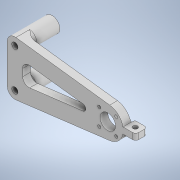
# Autodesk Inventor part: sensor_holder_1_mod
Saved by Autodesk Inventor 2020 (Build 240168000, 168)
## iProperties
Created: 2019-10-15
Part Number: sensor_holder_1_mod
Material: Generic
Document SubType Name: Modeling
Designer: psrob
Density: 1 g/cm^3
Appearance: Default
Author: psrob
Autodesk Inventor part; units mm, degrees
ref_plane "YZ Plane" through (0, 0, 0) normal (1, 0, 0) x (0, 1, 0)
ref_plane "XZ Plane" through (0, 0, 0) normal (0, 1, 0) x (-1, 0, 0)
ref_plane "XY Plane" through (0, 0, 0) normal (0, 0, 1) x (1, 0, 0)
sketch "Sketch1" plane through (0, 0, 0) normal (0, 0, 1) x (1, 0, 0)
  circle A0 centre (6, -12.5) radius 2
  circle A1 centre (6, 12.5) radius 2
  circle A2 centre (-10, -12.5) radius 2
  circle A3 centre (-10, 12.5) radius 2
  circle A4 centre (18, 0) radius 2.1
  circle A5 centre (28, 0) radius 2.1
  circle A6 centre (38, 0) radius 2.1
  circle A7 centre (50, 0) radius 6.5
  circle A8 centre (0, -12.5) radius 1.5
  circle A9 centre (0, 12.5) radius 1.5
  circle A10 centre (0, 0) radius 9
  line L0 (-6.52451, 22) -> (6.52451, 22)
  arc A11 (-8.148897, 20.972493) -> (-6.52451, 22) centre (-9.959763, 25.633047) ccw
  arc A12 (-8.148897, 20.972493) -> (-20.972493, 8.148897) centre (0, 0) ccw
  arc A13 (-22, 6.52451) -> (-20.972493, 8.148897) centre (-25.633047, 9.959763) ccw
  line L1 (-22, -6.52451) -> (-22, 6.52451)
  arc A14 (-20.972493, -8.148897) -> (-22, -6.52451) centre (-25.633047, -9.959763) ccw
  arc A15 (-20.972493, -8.148897) -> (-8.148897, -20.972493) centre (0, 0) ccw
  arc A16 (-6.52451, -22) -> (-8.148897, -20.972493) centre (-9.959763, -25.633047) ccw
  line L2 (6.52451, -22) -> (-6.52451, -22)
  arc A17 (8.148897, -20.972493) -> (6.52451, -22) centre (9.959763, -25.633047) ccw
  arc A18 (8.148897, -20.972493) -> (19.960204, -10.384615) centre (0, 0) ccw
  arc A19 (28.831406, -5) -> (19.960204, -10.384615) centre (28.831406, -15) ccw
  line L3 (28.831406, -5) -> (33.416876, -5)
  arc A20 (44.472292, -8.333333) -> (33.416876, -5) centre (33.416876, -25) ccw
  arc A21 (44.472292, -8.333333) -> (59.797959, -2) centre (50, 0) ccw
  arc A22 (33.416876, 5) -> (44.472292, 8.333333) centre (33.416876, 25) ccw
  line L4 (33.416876, 5) -> (28.831406, 5)
  arc A23 (19.960204, 10.384615) -> (28.831406, 5) centre (28.831406, 15) ccw
  arc A24 (19.960204, 10.384615) -> (8.148897, 20.972493) centre (0, 0) ccw
  arc A25 (6.52451, 22) -> (8.148897, 20.972493) centre (9.959763, 25.633047) ccw
  circle A26 centre (-10, -12.5) radius 5
  circle A27 centre (-10, 12.5) radius 5
  line L5 (66.5, 2) -> (66.5, -2)
  line L6 (66.5, 2) -> (59.797959, 2)
  arc A28 (59.797959, 2) -> (44.472292, 8.333333) centre (50, 0) ccw
  line L7 (59.797959, -2) -> (66.5, -2)
  dimension "d0" = 10
  dimension "d1" = 10
  constraints: 2 centre point, 2 coincident
  measures "d0" diameter of A26
  measures "d1" diameter of A27
extrude "Extrusion1" add sketch "Sketch1" along normal blind 20 contours A26 | A27
sketch "Sketch2" plane through (-10, -12.5, 20) normal (0, 0, 1) x (1, 0, 0)
  circle A0 centre (60, 12.5) radius 2.5
  circle A1 centre (60, 12.5) radius 10
  circle A2 centre (60, 12.5) radius 5
  circle A3 centre (0, 0) radius 5
  circle A4 centre (0, 0) radius 2
  circle A5 centre (0, 25) radius 5
  circle A6 centre (0, 25) radius 2
  line L0 (60, 12.5) -> (-0.617038, 4.96178)
  circle A7 centre (0, 0) radius 5
  line L1 (60, 12.5) -> (-0.617038, 20.03822)
  line L2 (0, 25) -> (-0.617038, 20.03822)
  line L3 (0, 0) -> (-0.617038, 4.96178)
  line L4 (61.234075, 2.576439) -> (0.617038, -4.96178)
  line L5 (0, 0) -> (0.617038, -4.96178)
  line L6 (60, 12.5) -> (61.234075, 2.576439)
  line L7 (61.234075, 22.423561) -> (0.617038, 29.96178)
  circle A8 centre (0, 25) radius 5
  line L8 (0, 25) -> (0.617038, 29.96178)
  line L9 (61.234075, 22.423561) -> (60, 12.5)
  point P0 (10, 12.5)
  point P1 (50.076439, 13.734075)
  point P2 (50.076439, 11.265925)
  point P3 (-0.617038, 4.96178)
  point P4 (0.617038, -4.96178)
  point P5 (0.617038, 29.96178)
  dimension "d4" = 20
  dimension "d5" = 10
  constraints: 20 end point, 6 perpendicular, 5 point on circle, 3 coincident, 2 centre point, 2 other
  measures "d4" diameter of A1
  measures "d5" diameter of A2
extrude "Extrusion2" add sketch "Sketch2" along normal blind 4 contours L9 A1 L6 A2 | A2 L1 A1 L9 | L6 A1 L0 A2 | A2 L0 A1 L1 | A1 L1 A5 L7 | L4 A3 L0 A1
sketch "Sketch3" plane through (0, 0, 20) normal (0, 0, 1) x (1, 0, 0)
  arc A0 (-10.617038, 7.53822) -> (-9.382962, 17.46178) centre (-10, 12.5) ccw
  arc A1 (-9.382962, 17.46178) -> (-10.617038, 7.53822) centre (-10, 12.5) ccw
  circle A2 centre (-10, 12.5) radius 2
  arc A3 (-9.382962, -17.46178) -> (-10.617038, -7.53822) centre (-10, -12.5) ccw
  arc A4 (-10.617038, -7.53822) -> (-9.382962, -17.46178) centre (-10, -12.5) ccw
  circle A5 centre (-10, -12.5) radius 2
  line L0 (-10, 12.5) -> (-15, 12.5)
  circle A6 centre (-10, 12.5) radius 5
  line L1 (-10, -12.5) -> (-15, -12.5)
  line L2 (-15, -12.5) -> (-15, 12.5)
  line L3 (-10, 12.5) -> (-5, 12.5)
  line L4 (-5, 12.5) -> (-5, -12.5)
  line L5 (-10, -12.5) -> (-5, -12.5)
  point P0 (0, 0)
  constraints: 12 end point, 4 point on circle, 3 perpendicular, 2 horizontal, 1 point on line
extrude "Extrusion3" add sketch "Sketch3" along normal blind 4 contours A1 L0 A2 L3 A0 | A0 L4 A3 A4 L2 A1 | L3 A2 L0 A1 A0 | L5 A5 L1 A4 A3 | A3 A4 L1 A5 L5
thicken "Thicken1" operation add thickness 1 both sides no extend neighbours yes toward (0, 0, -1) faces at (28.580011, -8.658994, 20)
thicken "Thicken2" operation add thickness 3 both sides no extend neighbours yes toward (-0.9953736, 0.0960805, 0) faces at (40.046264, 0.960805, 22.333333)
fillet "Fillet1" radius 4 2 edges at (-5, 6.8397, 21.5) (-5, -6.8397, 21.5)
fillet "Fillet2" radius 4 4 edges at (-10, 7.5, 19) (-6.2527, 15.8102, 19) (-6.2527, -15.8102, 19) (-10, -7.5, 19)
fillet "Fillet3" radius 2 2 edges at (37.0994, 1.6043, 21.5) (37.0994, -1.6043, 21.5)
sketch "Sketch4" plane through (0, 0, 0) normal (0, 1, 0) x (-1, 0, 0)
  line L0 (-51.234075, 19) -> (-51.234075, 19)
  line L1 (-51.234075, 19) -> (-51.234075, 24)
  line L2 (-51.234075, 24) -> (-51.234075, 24)
  line L3 (-51.234075, 19) -> (-51.234075, 24)
  line L4 (-51.234075, 24) -> (-60, 24)
  line L5 (-60, 24) -> (-68, 24)
  line L6 (-68, 24) -> (-68, 16.5)
  line L7 (-68, 16.5) -> (-60, 16.5)
  line L8 (-60, 16.5) -> (-60, 24)
  line L9 (-60, 24) -> (-57, 24)
  line L10 (-57, 24) -> (-57, 19)
  line L11 (-57, 19) -> (-60, 19)
  line L12 (-60, 19) -> (-60, 24)
  point P0 (0, 0)
  dimension "d17" = 8
  dimension "d18" = 7.5
  dimension "d19" = 3
  dimension "d20" = 5
  constraints: 16 end point, 4 parallel, 2 horizontal, 2 perpendicular
  measures "d17" distance of L7.end L6.end
  measures "d18" distance of L6.end L5.end
  measures "d19" distance of L10.end L11.end
  measures "d20" distance of L9.end L10.end
extrude "Extrusion4" add sketch "Sketch4" along normal mid plane 4
sketch "Sketch5" plane through (0, -2, 0) normal (0, -1, 0) x (1, 0, 0)
  line L0 (59.797959, 19) -> (59.797959, 24)
  line L1 (59.797959, 19) -> (60, 19)
  line L2 (60, 19) -> (60, 16.5)
  line L3 (60, 16.5) -> (68, 16.5)
  line L4 (68, 16.5) -> (68, 24)
  line L5 (68, 24) -> (59.797959, 24)
  line L6 (68, 24) -> (68, 16.5)
  line L7 (68, 20.25) -> (64, 20.25)
  circle A0 centre (64, 20.25) radius 1.5
  point P0 (0, 0)
  dimension "d23" = 4
  dimension "d24" = 3
  constraints: 2 end point, 1 centre point, 1 coincident, 1 horizontal, 1 midpoint
  measures "d23" distance of L7.start L7.end
  measures "d24" diameter of A0
extrude "Extrusion5" cut sketch "Sketch5" against normal blind 4 contours A0
fillet "Fillet4" radius 2 2 edges at (68, 0, 24) (68, 0, 16.5)
fillet "Fillet5" radius 1 2 edges at (60, 0, 19) (60, 0, 16.5)
sketch "Sketch6" plane through (-10, -12.5, 24) normal (0, 0, 1) x (1, 0, 0)
  line L0 (76, 14.5) -> (76, 10.5)
  line L1 (69.797959, 14.5) -> (76, 14.5)
  arc A0 (69.797959, 14.5) -> (61.234075, 22.423561) centre (60, 12.5) ccw
  line L2 (61.234075, 22.423561) -> (0.617038, 29.96178)
  arc A1 (0.617038, 29.96178) -> (-5, 25) centre (0, 25) ccw
  line L3 (-5, 25) -> (-5, 0)
  arc A2 (-5, 0) -> (0.617038, -4.96178) centre (0, 0) ccw
  line L4 (0.617038, -4.96178) -> (61.234075, 2.576439)
  arc A3 (61.234075, 2.576439) -> (69.797959, 10.5) centre (60, 12.5) ccw
  line L5 (76, 10.5) -> (69.797959, 10.5)
  circle A4 centre (60, 12.5) radius 5
  circle A5 centre (0, 25) radius 2
  circle A6 centre (0, 0) radius 2
  line L6 (9.49363, 18.780876) -> (44.040347, 14.484712)
  arc A7 (44.040347, 10.515288) -> (44.040347, 14.484712) centre (43.793532, 12.5) ccw
  line L7 (44.040347, 10.515288) -> (9.49363, 6.219124)
  arc A8 (5, 10.188548) -> (9.49363, 6.219124) centre (9, 10.188548) ccw
  line L8 (5, 10.188548) -> (5, 14.811452)
  arc A9 (9.49363, 18.780876) -> (5, 14.811452) centre (9, 14.811452) ccw
  circle A10 centre (60, 12.5) radius 6.5
  point P0 (10, 12.5)
  dimension "d29" = 13
  constraints: 1 centre point, 1 coincident
  measures "d29" diameter of A10
extrude "Extrusion6" cut sketch "Sketch6" against normal blind 10 contours A10
sketch "Sketch7" plane through (-10, -12.5, 24) normal (0, 0, 1) x (1, 0, 0)
  circle A0 centre (60, 12.5) radius 6.5
  line L0 (76, 14.5) -> (76, 10.5)
  line L1 (69.797959, 14.5) -> (76, 14.5)
  arc A1 (69.797959, 14.5) -> (61.234075, 22.423561) centre (60, 12.5) ccw
  line L2 (61.234075, 22.423561) -> (0.617038, 29.96178)
  arc A2 (0.617038, 29.96178) -> (-5, 25) centre (0, 25) ccw
  line L3 (-5, 25) -> (-5, 0)
  arc A3 (-5, 0) -> (0.617038, -4.96178) centre (0, 0) ccw
  line L4 (0.617038, -4.96178) -> (61.234075, 2.576439)
  arc A4 (61.234075, 2.576439) -> (69.797959, 10.5) centre (60, 12.5) ccw
  line L5 (76, 10.5) -> (69.797959, 10.5)
  circle A5 centre (0, 25) radius 2
  circle A6 centre (0, 0) radius 2
  line L6 (9.49363, 18.780876) -> (44.040347, 14.484712)
  arc A7 (44.040347, 10.515288) -> (44.040347, 14.484712) centre (43.793532, 12.5) ccw
  line L7 (44.040347, 10.515288) -> (9.49363, 6.219124)
  arc A8 (5, 10.188548) -> (9.49363, 6.219124) centre (9, 10.188548) ccw
  line L8 (5, 10.188548) -> (5, 14.811452)
  arc A9 (9.49363, 18.780876) -> (5, 14.811452) centre (9, 14.811452) ccw
  line L9 (65.5, 18) -> (65.5, 7)
  line L10 (65.5, 7) -> (54.5, 7)
  line L11 (54.5, 7) -> (54.5, 18)
  line L12 (54.5, 18) -> (65.5, 18)
  line L13 (65.5, 18) -> (54.5, 7) construction
  line L14 (65.5, 7) -> (54.5, 18) construction
  circle A10 centre (65.5, 18) radius 1
  circle A11 centre (65.5, 7) radius 1
  circle A12 centre (54.5, 18) radius 1
  circle A13 centre (54.5, 7) radius 1
  point P0 (10, 12.5)
  dimension "d32" = 11
  dimension "d33" = 11
  dimension "d34" = 2
  dimension "d35" = 2
  dimension "d36" = 2
  dimension "d37" = 2
  constraints: 12 end point, 4 centre point, 4 coincident, 2 midpoint, 2 parallel, 1 perpendicular, 1 vertical
  measures "d32" distance of L9.start L9.end
  measures "d33" distance of L9.end L10.end
  measures "d34" diameter of A10
  measures "d35" diameter of A11
  measures "d36" diameter of A12
  measures "d37" diameter of A13
extrude "Extrusion7" cut sketch "Sketch7" against normal blind 10 contours A10 L12 L9 | L9 L12 A10 | A11 L10 L9 | L9 L10 A11 | A12 L11 L12 | L12 L11 A12 | A13 L11 L10 | L10 L11 A13
thicken "Thicken3" operation add thickness 1.5 both sides no extend neighbours yes toward (-0.9870503, 0.1604113, 0) faces at (56.415827, -1.042673, 20.666667)
body "Solid1"
